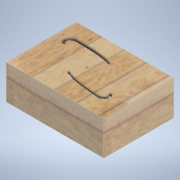
# Autodesk Inventor part: CigarBox
Saved by Autodesk Inventor 2021 (Build 250183000, 183)
## iProperties
Created: 2020-11-03
Part Number: CigarBox
Material: Wood (Maple)
Document SubType Name: Modeling
Designer: Cameron Chiaramonte
Density: 0.67 g/cm^3
Appearance: Natural Maple - Glossy Dark Tint
Author: Cameron Chiaramonte
Autodesk Inventor part; units mm, degrees
ref_plane "YZ Plane" through (0, 0, 0) normal (1, 0, 0) x (0, 1, 0)
ref_plane "XZ Plane" through (0, 0, 0) normal (0, 1, 0) x (-1, 0, 0)
sketch "Sketch1" plane through (0, 0, 0) normal (0, 1, 0) x (-1, 0, 0)
  line L0 (84.9737, 68.5674) -> (-162.6763, 68.5674)
  line L1 (-162.6763, 68.5674) -> (-162.6763, -109.2326)
  line L2 (-162.6763, -109.2326) -> (84.9737, -109.2326)
  line L3 (84.9737, -109.2326) -> (84.9737, 68.5674)
  point P0 (0, 0)
  dimension "d0" = 247.65
  dimension "d1" = 177.8
  constraints: 8 end point, 2 parallel, 1 horizontal, 1 perpendicular
  measures "d0" distance of L2.end L1.end
  measures "d1" distance of L1.end L0.end
extrude "Extrusion1" add sketch "Sketch1" along normal blind 4.7625
sketch "Sketch2" plane through (0, 4.7625, 0) normal (0, 1, 0) x (1, 0, 0)
  line L0 (-84.9737, 109.2326) -> (-84.9737, -68.5674) projected
  line L1 (162.6763, -68.5674) -> (162.6763, 109.2326) projected
  line L2 (-84.9737, -68.5674) -> (162.6763, -68.5674)
  line L3 (162.6763, -68.5674) -> (162.6763, -63.4874)
  line L4 (162.6763, -63.4874) -> (-84.9737, -63.4874)
  line L5 (-84.9737, -63.4874) -> (-84.9737, -68.5674)
  point P0 (0, 0)
  point P1 (-84.9737, -63.4874)
  dimension "d4" = 5.08
  constraints: 8 end point, 2 parallel, 1 horizontal, 1 perpendicular, 1 point on line
  measures "d4" distance of L3.end L2.end
extrude "Extrusion2" add sketch "Sketch2" along normal blind 82.55
sketch "Sketch3" plane through (0, 4.7625, 0) normal (0, 1, 0) x (1, 0, 0)
  line L0 (-84.9737, 109.2326) -> (-84.9737, -68.5674) projected
  line L1 (162.6763, -68.5674) -> (162.6763, 109.2326) projected
  line L2 (-84.9737, 109.2326) -> (162.6763, 109.2326)
  line L3 (162.6763, 109.2326) -> (162.6763, 104.1526)
  line L4 (162.6763, 104.1526) -> (-84.9737, 104.1526)
  line L5 (-84.9737, 104.1526) -> (-84.9737, 109.2326)
  point P0 (0, 0)
  point P1 (-84.9737, 104.1526)
  dimension "d7" = 5.08
  constraints: 8 end point, 2 parallel, 1 horizontal, 1 perpendicular, 1 point on line
  measures "d7" distance of L2.end L3.end
extrude "Extrusion3" add sketch "Sketch3" along normal blind 82.55
sketch "Sketch4" plane through (0, 4.7625, 0) normal (0, 1, 0) x (1, 0, 0)
  line L0 (-84.9737, -68.5674) -> (162.6763, -68.5674) projected
  line L1 (162.6763, 109.2326) -> (-84.9737, 109.2326) projected
  line L2 (-84.9737, -68.5674) -> (-79.8937, -68.5674)
  line L3 (-79.8937, -68.5674) -> (-79.8937, 109.2326)
  line L4 (-79.8937, 109.2326) -> (-84.9737, 109.2326)
  line L5 (-84.9737, 109.2326) -> (-84.9737, -68.5674)
  line L6 (162.6763, -68.5674) -> (157.5963, -68.5674)
  line L7 (157.5963, -68.5674) -> (157.5963, 109.2326)
  line L8 (157.5963, 109.2326) -> (162.6763, 109.2326)
  line L9 (162.6763, 109.2326) -> (162.6763, -68.5674)
  point P0 (0, 0)
  dimension "d10" = 5.08
  dimension "d11" = 5.08
  constraints: 16 end point, 4 parallel, 2 horizontal, 2 perpendicular, 2 point on line
  measures "d10" distance of L4.end L3.end
  measures "d11" distance of L7.end L8.end
extrude "Extrusion4" add sketch "Sketch4" along normal blind 82.55 contours L5 L1 L3 L0
sketch "Sketch5" plane through (0, 4.7625, 0) normal (0, 1, 0) x (1, 0, 0)
  line L0 (162.6763, 109.2326) -> (-84.9737, 109.2326) projected
  line L1 (-84.9737, -68.5674) -> (162.6763, -68.5674) projected
  line L2 (162.6763, 109.2326) -> (157.5963, 109.2326)
  line L3 (157.5963, 109.2326) -> (157.5963, -68.5674)
  line L4 (157.5963, -68.5674) -> (162.6763, -68.5674)
  line L5 (162.6763, -68.5674) -> (162.6763, 109.2326)
  point P0 (0, 0)
  dimension "d14" = 5.08
  constraints: 8 end point, 2 parallel, 1 horizontal, 1 perpendicular, 1 point on line
  measures "d14" distance of L4.end L3.end
extrude "Extrusion5" add sketch "Sketch5" along normal blind 82.55
sketch "Sketch6" plane through (-79.8937, 4.7625, -104.1526) normal (0, 0, 1) x (1, 0, 0)
  line L0 (-5.08, -4.7625) -> (-5.08, 82.55) projected
  line L1 (242.57, -4.7625) -> (242.57, 82.55) projected
  line L2 (-5.08, 82.55) -> (242.57, 82.55)
  line L3 (242.57, 82.55) -> (242.57, 76.2)
  line L4 (242.57, 76.2) -> (-5.08, 76.2)
  line L5 (-5.08, 76.2) -> (-5.08, 82.55)
  point P0 (79.8937, -4.7625)
  dimension "d17" = 6.35
  constraints: 8 end point, 2 parallel, 1 horizontal, 1 perpendicular, 1 point on line
  measures "d17" distance of L2.end L3.end
extrude "Extrusion6" add sketch "Sketch6" along normal blind 167.64
sketch "Sketch7" plane through (0, 0, 0) normal (0, -1, 0) x (1, 0, 0)
  point P0 (0, 0)
ref_plane "Work Plane1" through (0, 87.3125, 0) normal (0, 1, 0) x (1, 0, 0)
sketch "Sketch10" plane through (0, 87.3125, 0) normal (0, 1, 0) x (1, 0, 0)
  line L0 (-39.4156, 64.7377) -> (-51.6456, 64.7377) construction
  spline S0 degree 4 poles (-39.4156, 64.7377) (-51.6456, 64.7377) (-57.2894, 57.2798) (-57.2894, 50.8338) (-49.9984, 47.0841) knots 1 1 1 1 1 2 2 2 2 2
  line L1 (-51.6456, 64.7377) -> (-57.2894, 57.2798) construction
  line L2 (-57.2894, 57.2798) -> (-57.2894, 50.8338) construction
  line L3 (-57.2894, 50.8338) -> (-49.9984, 47.0841) construction
  line L4 (-46.1883, 71.1757) -> (-54.4299, 71.1757) construction
  spline S1 degree 4 poles (-46.1883, 71.1757) (-54.4299, 71.1757) (-64.3781, 58.0298) (-64.3781, 51.5837) (-58.1641, 45.0485) knots 1 1 1 1 1 2 2 2 2 2
  line L5 (-54.4299, 71.1757) -> (-64.3781, 58.0298) construction
  line L6 (-64.3781, 58.0298) -> (-64.3781, 51.5837) construction
  line L7 (-64.3781, 51.5837) -> (-58.1641, 45.0485) construction
  line L8 (-39.4156, 64.7377) -> (27.0232, 64.7377) construction
  spline S2 degree 2 poles (-39.4156, 64.7377) (27.0232, 64.7377) (46.0385, 54.8414) knots 1 1 1 2 2 2
  line L9 (27.0232, 64.7377) -> (46.0385, 54.8414) construction
  spline S3 degree 2 poles (-46.1883, 71.1757) (28.5034, 71.1757) (49.3836, 61.2115) knots 1 1 1 2 2 2
  line L10 (-46.1883, 71.1757) -> (28.5034, 71.1757) construction
  line L11 (28.5034, 71.1757) -> (49.3836, 61.2115) construction
  arc A0 (-58.1641, 45.0485) -> (-49.9984, 47.0841) centre (-54.6585, 48.3817) ccw
  arc A1 (46.0385, 54.8414) -> (49.3836, 61.2115) centre (47.6993, 58.0326) ccw
  line L12 (102.1246, -24.7938) -> (35.8412, -20.2518) construction
  spline S4 degree 2 poles (102.1246, -24.7938) (35.8412, -20.2518) (17.547, -9.0787) knots 1 1 1 2 2 2
  line L13 (35.8412, -20.2518) -> (17.547, -9.0787) construction
  spline S5 degree 2 poles (109.401, -29.8059) (34.884, -24.6997) (14.7339, -13.3314) knots 1 1 1 2 2 2
  line L14 (109.401, -29.8059) -> (34.884, -24.6997) construction
  line L15 (34.884, -24.6997) -> (14.7339, -13.3314) construction
  line L16 (120.9071, -12.1443) -> (113.8896, -7.905) construction
  spline S6 degree 4 poles (102.1246, -24.7938) (114.326, -25.6299) (120.4665, -18.5753) (120.9071, -12.1443) (113.8896, -7.905) knots 1 1 1 1 1 2 2 2 2 2
  line L17 (102.1246, -24.7938) -> (114.326, -25.6299) construction
  line L18 (114.326, -25.6299) -> (120.4665, -18.5753) construction
  line L19 (120.4665, -18.5753) -> (120.9071, -12.1443) construction
  line L20 (127.928, -13.3771) -> (122.1753, -6.4323) construction
  spline S7 degree 4 poles (109.401, -29.8059) (116.796, -30.3126) (127.4874, -19.8081) (127.928, -13.3771) (122.1753, -6.4323) knots 1 1 1 1 1 2 2 2 2 2
  line L21 (109.401, -29.8059) -> (116.796, -30.3126) construction
  line L22 (116.796, -30.3126) -> (127.4874, -19.8081) construction
  line L23 (127.4874, -19.8081) -> (127.928, -13.3771) construction
  arc A2 (122.1753, -6.4323) -> (113.8896, -7.905) centre (118.45, -9.5182) ccw
  arc A3 (17.547, -9.0787) -> (14.7339, -13.3314) centre (16.2173, -11.2559) ccw
  point P0 (0, 0)
  point P1 (0, 194.8532)
  constraints: 8 point on circle, 4 centre point, 4 point on line, 2 tangent, 26 other
extrude "Extrusion9" cut sketch "Sketch10" against normal blind 25.4
body "Solid1"
